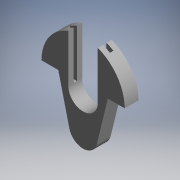
# Autodesk Inventor part: Contrap
Saved by Autodesk Inventor 2019.3 (Build 233278000, 278)
## iProperties
Part Number: Contrap
Material: Generic
Document SubType Name: Modeling
Designer: Usuario
Appearance: Default
Author: Usuario
Autodesk Inventor part; units mm, degrees
ref_plane "YZ Plane" through (0, 0, 0) normal (1, 0, 0) x (0, 1, 0)
ref_plane "XZ Plane" through (0, 0, 0) normal (0, 1, 0) x (-1, 0, 0)
ref_plane "XY Plane" through (0, 0, 0) normal (0, 0, 1) x (1, 0, 0)
sketch "Sketch1" plane through (0, 0, 0) normal (0, 0, 1) x (1, 0, 0)
  arc A0 (-12.7, 21.997) -> (12.7, 21.997) centre (0, 0) ccw
  arc A1 (-12.7, 23.8125) -> (12.7, 23.8125) centre (0, 0) ccw
  line L0 (-12.7, 21.997) -> (-12.7, 23.8125)
  line L1 (12.7, 21.997) -> (12.7, 23.8125)
  line L2 (-12.7, 23.8125) -> (12.7, 23.8125)
  arc A2 (-25.1613, -66.17) -> (25.1613, -66.17) centre (0, -59.9948) ccw
  line L3 (45.378, 16.2052) -> (25.1613, -66.17)
  line L4 (-45.378, 16.2052) -> (-25.1613, -66.17)
  line L5 (45.378, 16.2052) -> (76.2, 16.2052)
  line L6 (-45.378, 16.2052) -> (-76.2, 16.2052)
  line L7 (26.9875, 0) -> (26.9875, 87.4661)
  line L8 (-26.9875, 0) -> (-26.9875, 87.4661)
  arc A3 (76.2, 16.2052) -> (26.9875, 87.4661) centre (0, 16.2052) ccw
  arc A4 (-26.9875, 87.4661) -> (-76.2, 16.2052) centre (0, 16.2052) ccw
  dimension "d3" = 53.975
  dimension "d5" = 51.816
  dimension "d22" = 87.4661
  constraints: 18 end point, 12 point on circle, 5 centre point, 2 coincident, 2 vertical, 1 horizontal, 1 tangent
  measures "d3" diameter of A1
  measures "d5" diameter of A2
  measures "d22" distance of L8.start L8.end
extrude "Extrusion1" add sketch "Sketch1" along normal blind 25.4 contours A1 L7 A3 L5 L3 A2 L4 L6 A4 L8
sketch "Sketch2" plane through (-26.9875, 0, 0) normal (1, 0, 0) x (0, 0, -1)
  line L0 (0, 0) -> (0, 87.4661) projected
  line L1 (-25.4, 0) -> (-25.4, 87.4661) projected
  line L2 (-9.525, 87.4661) -> (-15.875, 87.4661)
  line L3 (-15.875, 0) -> (-9.525, 0)
  line L4 (0, 87.4661) -> (-25.4, 87.4661) construction
  line L5 (-12.7, 87.4661) -> (-12.7, 0) construction
  line L6 (0, 0) -> (-25.4, 0) construction
  line L7 (-9.525, 87.4661) -> (-9.525, 0)
  line L8 (-15.875, 87.4661) -> (-15.875, 0)
  dimension "d16" = 3.175
  dimension "d17" = 3.175
  constraints: 10 end point, 2 midpoint, 2 parallel, 1 horizontal, 1 perpendicular
  measures "d16" distance between parallel lines of L5 L7
  measures "d17" distance between parallel lines of L5 L8
extrude "Extrusion2" cut sketch "Sketch2" against normal blind 12.7 and the other way blind 66.675
body "Solid1"
